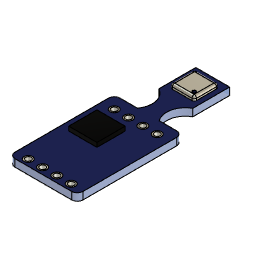
Temperature, Humidity, Pressure Sensor (Autodesk Fusion 360 design; units mm, degrees)
Autodesk Fusion 360 part; units mm, degrees
note: some values were not read from the file. Set by a fixed rule: which face or edge a step refers to.
sketch "Sketch1" plane through (0, 0, 0) normal (0, 0, 1) x (1, 0, 0)
  line L0 (5.0325, -15.0115) -> (-5.0325, -15.0115)
  line L1 (-6.0325, -14.0115) -> (-6.0325, 2.5985)
  line L2 (-6.0325, 15.0115) -> (6.0325, 15.0115)
  line L3 (6.0325, 2.5985) -> (6.0325, -14.0115)
  line L4 (6.0325, -15.0115) -> (-6.0325, 15.0115) construction
  line L5 (-6.0325, -15.0115) -> (6.0325, 15.0115) construction
  line L6 (0, 15.0115) -> (0, -15.0115) construction
  circle A0 centre (-3.81, -13.8715) radius 0.75
  circle A1 centre (-3.81, -13.8715) radius 0.5
  circle A2 centre (-1.27, -13.8715) radius 0.75
  circle A3 centre (-1.27, -13.8715) radius 0.5
  circle A4 centre (1.27, -13.8715) radius 0.75
  circle A5 centre (1.27, -13.8715) radius 0.5
  circle A6 centre (3.81, -13.8715) radius 0.75
  circle A7 centre (3.81, -13.8715) radius 0.5
  circle A8 centre (-3.81, 1.3685) radius 0.75
  circle A9 centre (-3.81, 1.3685) radius 0.5
  circle A10 centre (-1.27, 1.3685) radius 0.75
  circle A11 centre (-1.27, 1.3685) radius 0.5
  circle A12 centre (1.27, 1.3685) radius 0.75
  circle A13 centre (1.27, 1.3685) radius 0.5
  circle A14 centre (3.81, 1.3685) radius 0.75
  circle A15 centre (3.81, 1.3685) radius 0.5
  line L7 (-5.0325, 3.5985) -> (5.0325, 3.5985)
  line L8 (-1.27, 3.5985) -> (-1.27, 8.4787) construction
  line L9 (1.27, 3.5985) -> (1.27, 8.4787) construction
  line L10 (1.27, 8.4787) -> (3, 8.4787) construction
  line L11 (3, 8.4787) -> (3, 15.0115)
  line L12 (-1.27, 8.4787) -> (-3, 8.4787) construction
  line L13 (-3, 8.4787) -> (-3, 15.0115)
  arc A16 (3, 8.4787) -> (1.9309, 3.5985) centre (4.566, 5.5785) ccw
  arc A17 (-1.9309, 3.5985) -> (-3, 8.4787) centre (-4.566, 5.5785) ccw
  arc A18 (-5.0325, 3.5985) -> (-6.0325, 2.5985) centre (-5.0325, 2.5985) ccw
  arc A19 (6.0325, 2.5985) -> (5.0325, 3.5985) centre (5.0325, 2.5985) ccw
  arc A20 (5.0325, -15.0115) -> (6.0325, -14.0115) centre (5.0325, -14.0115) ccw
  arc A21 (-6.0325, -14.0115) -> (-5.0325, -15.0115) centre (-5.0325, -14.0115) ccw
  line L14 (2.135, 9.6001) -> (-2.135, 9.6001)
  line L15 (-2.135, 9.6001) -> (-2.135, 13.9291)
  line L16 (-2.135, 13.9291) -> (2.135, 13.9291)
  line L17 (2.135, 13.9291) -> (2.135, 9.6001)
  line L18 (2.135, 9.6001) -> (-2.135, 13.9291) construction
  line L19 (-2.135, 9.6001) -> (2.135, 13.9291) construction
  circle A22 centre (1.2975, 10.4492) radius 0.2957
  line L20 (-4.5, -1) -> (0.5, -1)
  line L21 (0.5, -1) -> (0.5, -6)
  line L22 (0.5, -6) -> (-4.5, -6)
  line L23 (-4.5, -6) -> (-4.5, -1)
  point P0 (0, 11.7646)
  dimension "d1" = 30.023
  dimension "d2" = 12.065
  dimension "d3" = 1.5
  dimension "d4" = 1
  dimension "d5" = 3.81
  dimension "d8" = 7.62
  dimension "d9" = 15.24
  dimension "d10" = 2.23
  dimension "d11" = 2.54
  dimension "d12" = 1
  dimension "d13" = 1
  dimension "d14" = 1
  dimension "d15" = 1
  dimension "d16" = 2.2225
  dimension "d29" = 5
  dimension "d30" = 5
  constraint perpendicular L0 L1
  constraint parallel L0 L2
  constraint parallel L1 L3
  constraint horizontal L0
  constraint coincident L4 origin
  constraint coincident L5 origin
  constraint midpoint L2 L6.start
  constraint concentric A0 A1
  constraint perpendicular L3 L7
  constraint coincident L7 L8.start
  constraint perpendicular L7 L8
  constraint coincident L7 L9.start
  constraint perpendicular L7 L9
  constraint perpendicular L9 L10
  constraint coincident L2 L11.end
  constraint perpendicular L2 L11
  constraint symmetric L6 L9.end L8.end
  constraint symmetric L6 L10.end L12.end
  constraint symmetric L6 L11.end L13.end
  constraint tangent L9 A16
  constraint coincident L7 A16.end
  constraint symmetric L6 A16.end A17.start
  constraint symmetric L6 A16 A17
  constraint tangent L1 A18
  constraint tangent L7 A18
  constraint coincident L2.end L3
  constraint tangent L3 A19
  constraint tangent L7 A19
  constraint coincident L0 L6.end
  constraint coincident L4.start L0
  constraint coincident L4.start L3
  constraint tangent L0 A20
  constraint tangent L3 A20
  constraint coincident L5.start L0
  constraint coincident L5.start L1
  constraint tangent L0 A21
  constraint tangent L1 A21
  constraint perpendicular L14 L15
  constraint parallel L14 L16
  constraint parallel L15 L17
  constraint horizontal L14
  constraint coincident L18 P0
  constraint coincident L19 P0
  constraint coincident L6 P0
  constraint coincident L18 A22.centre
  constraint horizontal L20
  constraint vertical L21
  constraint horizontal L22
  constraint vertical L23
  measures "d1" distance of L0 L2
  measures "d2" distance of L1 L3
  measures "d3" diameter of A0
  measures "d4" diameter of A1
  measures "d5" distance of L6 A0.centre
  measures "d10" distance of A10.centre L7
  measures "d11" distance of L8 L9
  measures "d12" radius of A18
  measures "d13" radius of A19
  measures "d14" radius of A20
  measures "d15" radius of A21
  measures "d16" distance of L3 A6.centre
  measures "d29" distance of L20.start L20.end
  measures "d30" distance of L20.start L22.end
extrude "Extrude1" add sketch "Sketch1" along normal blind 1.3 contours L0 L1 L3 L7 A18 A19 A20 A21 | L2 L7 L11 L13 A16 A17 | L14 L15 L16 L17 | A22 | L20 L21 L22 L23 makes body 1
extrude "Extrude1'" add sketch "Sketch1" along normal up to surface (1.3 mm away) separate body contours A0 | A2 | A4 | A6 | A8 | A10 | A12 | A14 makes body 2 at (2.0191, 1.3311, 0.8667) makes body 3 at (-0.5209, -13.9089, 0.8667) makes body 4 at (0.5237, -13.9462, 0.8667) makes body 5 at (-0.5209, 1.3311, 0.8667) makes body 6 at (4.5591, 1.3311, 0.8667) makes body 7 at (-4.5563, -13.9462, 0.8667) makes body 8 at (4.5591, -13.9089, 0.8667) makes body 9 at (-3.0609, 1.3311, 0.8667) in component "Component"
extrude "Extrude2" add sketch "Sketch1" along normal blind 0.75 from surface at 1.3 separate body contours L14 L15 L16 L17 | A22 makes body 10
fillet "Fillet1" radius 0.4 8 edges at (2.135, 11.7646, 2.05) (2.135, 9.6001, 1.675) (0, 9.6001, 2.05) (0, 13.9291, 2.05) (2.135, 13.9291, 1.675) (-2.135, 13.9291, 1.675) (-2.135, 11.7646, 2.05) (-2.135, 9.6001, 1.675) on bodies 10
shell "Shell1" thickness 0.1 removed faces 1 at (0.7117, 11.1764, 1.3) on bodies 10
extrude "Extrude3" cut sketch "Sketch1" along normal up to surface (0.1 mm away) from surface at 1.95 contours A22 bodies 10
extrude "Extrude1''" add sketch "Sketch1" along normal blind 0.75 from surface at 1.3 separate body contours L20 L21 L22 L23 makes body 11 in component "Component'"
component "Component" placed x (1, 0, 0) y (0, 1, 0) z (0, 0, 1) at (0, 0, 0)
component "Component'" placed x (1, 0, 0) y (0, 1, 0) z (0, 0, 1) at (0, 0, 0)
